Autodesk Fusion 360 part; units mm, degrees
(part 3 of 3)
  spline S314 degree 3 poles (-31.4258, 46.0917) (-30.862, 46.1019) (-30.587, 45.6049) (-30.8545, 45.1043) knots 0 0 0 0 1 1 1 1
  spline S315 degree 3 poles (-30.8545, 45.1043) (-30.9345, 44.9544) (-31.0718, 44.9552) (-31.206, 44.9555) knots 0 0 0 0 1 1 1 1
  spline S316 degree 3 poles (-31.206, 44.9555) (-32.1079, 44.9577) (-33.0098, 44.9638) (-33.944, 44.9787) knots 0 0 0 0 1 1 1 1
  spline S317 degree 3 poles (-49.7648, 46.0737) (-49.7338, 45.8714) (-49.8388, 45.6725) (-49.6485, 45.5114) knots 0 0 0 0 1 1 1 1
  spline S318 degree 3 poles (-49.6485, 45.5114) (-49.4348, 45.6603) (-49.5439, 45.875) (-49.5205, 46.0517) knots 0 0 0 0 1 1 1 1
  spline S319 degree 3 poles (-49.5205, 46.0517) (-49.5044, 46.1733) (-49.5171, 46.2985) (-49.5093, 46.4216) knots 0 0 0 0 1 1 1 1
  spline S320 degree 3 poles (-49.5093, 46.4216) (-49.5016, 46.5425) (-49.4146, 46.5916) (-49.3087, 46.5996) knots 0 0 0 0 1 1 1 1
  spline S321 degree 3 poles (-49.3087, 46.5996) (-49.1829, 46.6091) (-49.1312, 46.5206) (-49.1251, 46.4136) knots 0 0 0 0 1 1 1 1
  spline S322 degree 3 poles (-49.1251, 46.4136) (-49.1152, 46.2413) (-49.1209, 46.0681) (-49.1171, 45.8954) knots 0 0 0 0 1 1 1 1
  spline S323 degree 3 poles (-49.1171, 45.8954) (-49.1129, 45.7035) (-49.1659, 45.4889) (-48.8889, 45.4187) knots 0 0 0 0 1 1 1 1
  spline S324 degree 3 poles (-48.8889, 45.4187) (-48.7852, 45.3925) (-48.7964, 45.2833) (-48.8106, 45.1977) knots 0 0 0 0 1 1 1 1
  spline S325 degree 3 poles (-48.8106, 45.1977) (-48.8262, 45.1032) (-48.9068, 45.0949) (-48.9815, 45.0947) knots 0 0 0 0 1 1 1 1
  spline S326 degree 3 poles (-48.9815, 45.0947) (-49.3398, 45.0934) (-49.698, 45.0924) (-50.0562, 45.0964) knots 0 0 0 0 1 1 1 1
  spline S327 degree 3 poles (-50.0562, 45.0964) (-50.3384, 45.0996) (-50.2283, 45.4152) (-50.3843, 45.5222) knots 0 0 0 0 1 1 1 1
  spline S328 degree 3 poles (-50.3843, 45.5222) (-50.4048, 45.5066) (-50.4307, 45.4967) (-50.4401, 45.4784) knots 0 0 0 0 1 1 1 1
  spline S329 degree 3 poles (-50.4401, 45.4784) (-50.5277, 45.3085) (-50.5084, 45.0225) (-50.8289, 45.1027) knots 0 0 0 0 1 1 1 1
  spline S330 degree 3 poles (-50.8289, 45.1027) (-51.1248, 45.1769) (-50.9685, 45.4261) (-50.9998, 45.5984) knots 0 0 0 0 1 1 1 1
  spline S331 degree 3 poles (-50.9998, 45.5984) (-51.0215, 45.718) (-51.0041, 45.8447) (-51.0038, 45.9682) knots 0 0 0 0 1 1 1 1
  spline S332 degree 3 poles (-51.0038, 45.9682) (-51.0023, 46.5601) (-50.9158, 46.6578) (-50.3347, 46.5803) knots 0 0 0 0 1 1 1 1
  spline S333 degree 3 poles (-50.3347, 46.5803) (-50.1667, 46.5579) (-49.9942, 46.5809) (-49.8296, 46.5371) knots 0 0 0 0 1 1 1 1
  spline S334 degree 3 poles (-49.8296, 46.5371) (-49.7213, 46.402) (-49.7828, 46.248) (-49.7648, 46.0737) knots 0 0 0 0 1 1 1 1
extrude "Extrude7" cut sketch "Sketch10" against normal blind 2 contours S0 S1 S2 S3 S4 S5 S6 S7 S8 S9 S10 S11 S12 S13 S14 S15 S16 S17 S18 S19 S20 S21 S22 S23 S24 S25 S26 S27 S28 S29 S30 S31 S32 S33 S34 S35 S36 S37 S38 S39 S40 S41 S42 S43 S44 S45 S46 S47 S48 S49 S50 S51 S52 | S53 S54 S55 S56 S57 S58 S59 S60 S61 S62 S63 S64 S65 S66 S67 S68 S69 S70 S71 S72 S73 S74 S75 S76 S77 S78 S79 S80 S81 S82 S83 S84 S85 S86 S87 | S88 S89 S90 S91 S92 S93 S94 S95 S96 S97 S98 S99 S100 S101 S102 | S103 S104 S105 S106 S107 S108 S109 | S110 S111 S112 S113 S114 S115 S116 S117 S118 S119 | S132 S133 S134 S135 S136 S137 S138 S139 S140 S141 S142 S143 S144 S145 S146 S147 S148 S149 S150 S151 S152 | S160 S161 S162 S163 S164 S165 S166 S167 | S175 S176 S177 S178 S179 S180 S181 S182 S183 S184 S185 S186 S187 S188 S189 S190 S191 S192 S193 S194 | S195 S196 S197 S198 S199 S200 S201 S202 | S211 S212 S213 S214 S215 S216 S217 S218 S219 S220 S221 S222 S223 | S224 S225 S226 S227 S228 S229 S230 S231 S232 S233 S234 S235 S236 | S237 S238 S239 S240 S241 S242 S243 S244 S245 S246 S247 S248 S249 S250 S251 S252 S253 | S254 S255 S256 S257 S258 S259 S260 S261 S262 | S269 S270 S271 S272 S273 S274 S275 S276 S277 S278 S279 S280 S281 S282 | S287 S288 S289 S290 S291 S292 S293 S294 S295 S296 S297 S298 S299 S300 S301 S302 S303 S304 S305 | S306 S307 S308 S309 S310 S311 S312 S313 S314 S315 S316 | S317 S318 S319 S320 S321 S322 S323 S324 S325 S326 S327 S328 S329 S330 S331 S332 S333 S334
